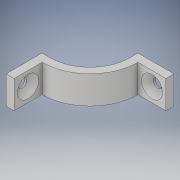
# Autodesk Inventor part: wiresHolder
Saved by Autodesk Inventor 2019 (Build 230136000, 136)
## iProperties
Created: 2019-08-23
Part Number: wiresHolder
Material: Generic
Document SubType Name: Modeling
Designer: fablab
Density: 1 g/cm^3
Appearance: Default
Author: fablab
Autodesk Inventor part; units mm, degrees
ref_plane "YZ Plane" through (0, 0, 0) normal (1, 0, 0) x (0, 1, 0)
ref_plane "XZ Plane" through (0, 0, 0) normal (0, 1, 0) x (-1, 0, 0)
ref_plane "XY Plane" through (0, 0, 0) normal (0, 0, 1) x (1, 0, 0)
sketch "Sketch3" plane through (0, 0, 0) normal (0, 1, 0) x (-1, 0, 0)
  arc A0 (0, 10) -> (-10, 0) centre (0, 0) ccw
  arc A1 (0, 12) -> (-12, 0) centre (0, 0) ccw
  line L0 (0, 10) -> (2, 10)
  line L1 (2, 10) -> (2, 19)
  line L2 (2, 19) -> (0, 19)
  line L3 (0, 19) -> (0, 10)
  line L4 (-10, 0) -> (-19, 0)
  line L5 (-19, 0) -> (-19, -2)
  line L6 (-19, -2) -> (-10, -2)
  line L7 (-10, -2) -> (-10, 0)
  line L8 (0, 12) -> (0, 10)
  line L9 (-10, 0) -> (-12, 0)
  dimension "d10" = 10
  dimension "d11" = 12
  dimension "d12" = 2
  dimension "d13" = 9
  dimension "d14" = 9
  dimension "d15" = 2
  constraints: 20 end point, 4 parallel, 4 point on circle, 2 centre point, 2 coincident, 2 collinear, 2 horizontal, 2 perpendicular
  measures "d10" radius of A0
  measures "d11" radius of A1
  measures "d12" distance of L2.end L1.end
  measures "d13" distance of L1.end L0.end
  measures "d14" distance of L6.end L5.end
  measures "d15" distance of L5.end L4.end
extrude "Extrusion2" add sketch "Sketch3" along normal blind 7
sketch "Sketch4" plane through (0, 0, 19) normal (1, 0, 0) x (0, 0, -1)
  line L0 (0, 0) -> (0, 7) projected
  line L1 (0, 3.5) -> (7, 3.5) construction
  line L2 (7, 0) -> (7, 7) projected
  line L3 (7, 0) -> (7, 7) construction
  line L4 (0, 7) -> (7, 7) construction
  line L5 (0, 0) -> (0, 7) construction
  line L6 (0, 0) -> (7, 0) construction
  line L7 (9, 7) -> (0, 7) construction
  line L8 (3.5, 7) -> (3.5, 3.5) construction
  circle A0 centre (3.5, 3.5) radius 1.15
  point P0 (19, 0)
  dimension "d18" = 2.3
  constraints: 4 end point, 3 midpoint, 1 centre point, 1 coincident, 1 point on line
  measures "d18" diameter of A0
extrude "Extrusion3" cut sketch "Sketch4" against normal blind 2
chamfer "Chamfer1" distance 1.5 angle 45 1 edges at (0, 3.5, 16.65)
sketch "Sketch6" plane through (12, 0, 0) normal (0, 0, 1) x (1, 0, 0)
  line L0 (7, 0) -> (7, 7) projected
  line L1 (7, 3.5) -> (0.0163, 3.5) construction
  line L2 (0, 7) -> (7, 7) projected
  line L3 (3.5, 7) -> (3.5082, 3.5) construction
  circle A0 centre (3.5082, 3.5) radius 1.15
  point P0 (-12, 0)
  dimension "d24" = 2.3
  constraints: 4 end point, 3 midpoint, 1 centre point, 1 coincident, 1 horizontal
  measures "d24" diameter of A0
extrude "Extrusion4" cut sketch "Sketch6" against normal blind 2
chamfer "Chamfer2" distance 1.5 angle 45 1 edges at (14.3582, 3.5, 0)
body "Solid2"
